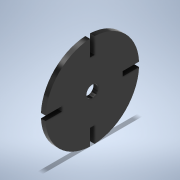
# Autodesk Inventor part: Encoder_Disk
Saved by Autodesk Inventor 2020 (Build 240168000, 168)
## iProperties
Created: 2020-07-31
Part Number: Encoder_Disk
Material: Generic
Document SubType Name: Modeling
Designer: Abbas
Density: 1 g/cm^3
Appearance: Default
Author: Abbas
Autodesk Inventor part; units mm, degrees
ref_plane "YZ Plane" through (0, 0, 0) normal (1, 0, 0) x (0, 1, 0)
ref_plane "XZ Plane" through (0, 0, 0) normal (0, 1, 0) x (-1, 0, 0)
ref_plane "XY Plane" through (0, 0, 0) normal (0, 0, 1) x (1, 0, 0)
sketch "Sketch1" plane through (0, 0, 0) normal (1, 0, 0) x (0, 1, 0)
  circle A0 centre (0, 0) radius 2.5
  line L0 (19.975, 1) -> (13, 1)
  line L1 (13, 1) -> (13, -1)
  line L2 (13, -1) -> (19.975, -1)
  line L3 (-1, 19.975) -> (-1, 13)
  line L4 (-1, 13) -> (1, 13)
  line L5 (1, 13) -> (1, 19.975)
  line L6 (-19.975, -1) -> (-13, -1)
  line L7 (-13, -1) -> (-13, 1)
  line L8 (-13, 1) -> (-19.975, 1)
  line L9 (1, -19.975) -> (1, -13)
  line L10 (1, -13) -> (-1, -13)
  line L11 (-1, -13) -> (-1, -19.975)
  arc A1 (19.975, 1) -> (1, 19.975) centre (0, 0) ccw
  arc A2 (1, -19.975) -> (19.975, -1) centre (0, 0) ccw
  arc A3 (-1, 19.975) -> (-19.975, 1) centre (0, 0) ccw
  arc A4 (-19.975, -1) -> (-1, -19.975) centre (0, 0) ccw
  dimension "d1" = 5
  dimension "d6" = 360
  constraints: 24 end point, 8 point on circle, 5 centre point, 2 coincident, 1 horizontal, 1 parallel, 1 perpendicular, 29 other
  measures "d1" diameter of A0
extrude "Extrusion1" add sketch "Sketch1" along normal blind 2
body "Solid1"
